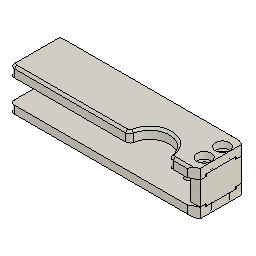
Summit (Autodesk Fusion 360 design; units mm, degrees)
Autodesk Fusion 360 part; units mm, degrees
sketch "Faceplate_Profile" plane through (0, 0, 0) normal (0, 0, 1) x (1, 0, 0)
  line L0 (0, 0) -> (85, 0)
  line L1 (85, 0) -> (85, 23)
  line L2 (85, 23) -> (0, 23)
  line L3 (0, 23) -> (0, 0)
  arc A0 (72.75, 0) -> (54.75, 0) centre (63.75, 0.1978) ccw
  line L4 (63.75, 0.1978) -> (63.75, 9.2) construction
  circle A1 centre (88, 11.5) radius 12 construction
  line L5 (85, 11.5) -> (88, 11.5) construction
  line L6 (80.7138, 21.0347) -> (80.7138, 1.9653)
  line L7 (80.7138, 1.9653) -> (89.4835, -4.7363) construction
  line L8 (80.7138, 21.0347) -> (88.5708, 27.0388) construction
  arc A2 (80.7138, 21.0347) -> (80.7138, 1.9653) centre (88, 11.5) ccw
  line L9 (84.2138, 26.5305) -> (84.2138, -3.5305) construction
  arc A3 (84.2138, 26.5305) -> (84.2138, -3.5305) centre (88, 11.5) ccw construction
  line L10 (72.5, 23) -> (72.5, 0) construction
  line L11 (80.7138, 1.9653) -> (72.5, 1.9653)
  line L12 (72.5, 1.9653) -> (72.5, 21.0347)
  line L13 (72.5, 21.0347) -> (80.7138, 21.0347)
  line L14 (80.7138, 21.0347) -> (80.7138, 1.9653)
  circle A4 centre (70.5, 11.5) radius 2
  line L15 (80.7138, 21.0347) -> (85, 21.0347)
  line L16 (80.7138, 1.9653) -> (85, 1.9653)
  dimension "d12" = 85
  dimension "d13" = 23
  dimension "d14" = 9.2
  dimension "d16" = 63.75
  dimension "d17" = 18
  dimension "d42" = 24
  dimension "d43" = 3
  dimension "d44" = 3.5
  dimension "d45" = 4
  constraint horizontal L0
  constraint vertical L1
  constraint horizontal L2
  constraint vertical L3
  constraint coincident L0.start L3.end
  constraint coincident L0 A0.end
  constraint coincident L0 A0.start
  constraint coincident A0.centre L4.start
  constraint midpoint A0 L4.end
  constraint midpoint L1 L5.start
  constraint coincident A1.centre L5.end
  constraint horizontal L5
  constraint coincident A1 L6.start
  constraint coincident A1 L6.end
  constraint vertical L6
  constraint tangent A1 L8
  constraint tangent A1 L7
  constraint tangent L7 A2
  constraint coincident L2 L10.start
  constraint coincident L0 L10.end
  constraint perpendicular L0 L10
  constraint horizontal L11
  constraint vertical L12
  constraint horizontal L13
  constraint vertical L14
  constraint tangent L12 A4
  constraint coincident L1 L15.end
  constraint perpendicular L1 L15
  constraint perpendicular L6 L16
  measures "d12" distance of L0.start L0.end
  measures "d13" distance of L0.start L2.end
  measures "d14" distance of L0 L4.end
  measures "d16" horizontal distance of L0.start A0.centre
  measures "d17" distance of A0.end A0.start
  measures "d42" diameter of A1
  measures "d43" distance of L1 A1.centre
  measures "d45" diameter of A4
extrude "Extrude1" add sketch "Faceplate_Profile" along normal blind 4.6 contours A4 | L0 L1 L2 L3 A0 L12 L13 L15 | L0 L1 A0 L11 L16 | A0 A2 L11 L12 L13 | L1 L6 L14 L15 L16 | L6 A2 L14 makes body 1 in component "Plate_Top"
extrude "Extrude1'" add sketch "Faceplate_Profile" against normal blind 4.6 from surface at -10.8 separate body contours A4 | L0 L1 L2 L3 A0 L12 L13 L15 | L0 A0 L11 L12 | L0 L1 A0 L11 L16 | A0 A2 L11 L12 L13 | A0 L11 L12 | L1 L6 L14 L15 L16 | L6 A2 L14 makes body 2 in component "Plate_Bottom"
extrude "Extrude1''" add sketch "Faceplate_Profile" against normal up to surface (10.8 mm away) separate body contours A4 | L1 L6 L14 L15 L16 | L6 A2 L14 makes body 3 at (76.9486, 16.1761, -7.2) makes body 4 at (69.1766, 12.9996, -7.2) in component "Ring_Holder"
sketch "Holder things" plane through (0, 0, -10.8) normal (0, 0, 1) x (-1, 0, 0) in component "Ring_Holder"
  line L0 (-85, 0) -> (-85, -23)
  line L1 (-85, -23) -> (0, -23)
  line L2 (0, -23) -> (0, 0)
  line L3 (0, 0) -> (-85, 0)
  arc A0 (-80.7138, -21.0347) -> (-80.7138, -1.9653) centre (-88, -11.5) ccw
  line L4 (-80.7138, -1.9653) -> (-85, -1.9653)
  line L5 (-85, -1.9653) -> (-85, -21.0347)
  line L6 (-85, -21.0347) -> (-80.7138, -21.0347)
  circle A1 centre (-70.5, -11.5) radius 2
  line L7 (0, 0) -> (-85, 0)
  line L8 (-85, 0) -> (-85, -23)
  line L9 (0, -23) -> (0, 0)
  line L10 (-85, -23) -> (0, -23)
  line L11 (-78.0788, -18.2506) -> (-78.0788, -4.7494)
  line L12 (-78.0788, -4.7494) -> (-85, -4.7494)
  line L13 (-85, -4.7494) -> (-85, -18.2506)
  line L14 (-85, -18.2506) -> (-78.0788, -18.2506)
  circle A2 centre (-81.5394, -7.2929) radius 1.5
  circle A3 centre (-81.5394, -15.7071) radius 1.5
  line L15 (-81.5394, -7.2929) -> (-81.5394, -15.7071) construction
  line L16 (-78.0788, -11.5) -> (-85, -11.5) construction
  circle A4 centre (-70.5, -11.5) radius 1.5
  point P0 (-70.5, -11.5)
  dimension "d48" = 3
  dimension "d49" = 3
  dimension "d50" = 3
  constraint perpendicular L11 L12
  constraint parallel L11 L13
  constraint parallel L12 L14
  constraint coincident A0 L11.end
  constraint vertical L11
  constraint coincident A0 L11.start
  constraint coincident A2.centre L15.start
  constraint coincident A3.centre L15.end
  constraint vertical L15
  constraint midpoint L11 L16.start
  constraint midpoint L5 L16.end
  constraint midpoint L15 L16
  constraint coincident P0 A1.centre
  measures "d48" diameter of A2
  measures "d49" diameter of A3
  measures "d50" diameter of A4
extrude "Extrude2" cut sketch "Holder things" along normal blind -1 and the other way blind 0 contours L0 L5 L8 L11 L12 L13 L14 | A2 | A3 bodies 2 in component "Plate_Bottom"
extrude "Extrude2'" cut sketch "Holder things" along normal blind 1 from surface at 10.8 contours L0 L5 L8 L11 L12 L13 L14 | A2 | A3 bodies 1 in component "Plate_Top"
extrude "Extrude2''" add sketch "Holder things" against normal blind 1 contours L0 L5 L8 L11 L12 L13 L14 bodies 3 in component "Ring_Holder"
extrude "Extrude3" add sketch "Holder things" along normal blind 1 from surface at 10.8 contours L0 L5 L8 L11 L12 L13 L14 bodies 3 in component "Ring_Holder"
move_face "OffsetFaces1" offset -0.2 3 faces at (82.6929, 18.2506, -11.1333) (80.3859, 4.7494, -11.1333) (78.0788, 13.7502, -11.1333) on bodies 2 in component "Plate_Bottom"
move_face "OffsetFaces1'" offset -0.2 3 faces at (78.0788, 13.7502, 0.3333) (82.6929, 18.2506, 0.3333) (80.3859, 4.7494, 0.3333) on bodies 1 in component "Plate_Top"
sketch "D_plate_bores" plane through (0, 0, 4.6) normal (0, 0, 1) x (-1, 0, 0) in component "Ring_Holder"
  line L0 (-85, 0) -> (-85, -23)
  line L1 (-85, -23) -> (0, -23)
  line L2 (0, -23) -> (0, 0)
  line L3 (0, 0) -> (-54.75, 0)
  arc A0 (-72.75, 0) -> (-54.75, 0) centre (-63.75, -0.1978) ccw
  line L4 (-72.75, 0) -> (-85, 0)
  circle A1 centre (-70.5, -11.5) radius 2
  circle A2 centre (-70.5, -11.5) radius 2
  line L5 (-85, -4.7494) -> (-85, -18.2506)
  line L6 (-85, -18.2506) -> (-78.0788, -18.2506)
  line L7 (-78.0788, -18.2506) -> (-78.0788, -4.7494)
  line L8 (-78.0788, -4.7494) -> (-85, -4.7494)
  circle A3 centre (-81.5394, -15.7071) radius 1.5
  circle A4 centre (-81.5394, -7.2929) radius 1.5
hole "Hole1" at (81.5394, 7.2929, 4.6) at (81.5394, 15.7071, 4.6) direction (0, 0, -1) diameter 3.4 depth 19 tip angle 180 counterbore diameter 6.5 counterbore depth 3 bodies 1 in component "Plate_Top"
hole "Hole1'" at (81.5394, 7.2929, 4.6) at (81.5394, 15.7071, 4.6) direction (0, 0, -1) diameter 3.4 depth 19 tip angle 180 counterbore diameter 6.5 counterbore depth 3 bodies 2 in component "Plate_Bottom"
hole "Hole1''" at (81.5394, 7.2929, 4.6) at (81.5394, 15.7071, 4.6) direction (0, 0, -1) diameter 3.4 depth 19 tip angle 180 counterbore diameter 6.5 counterbore depth 3 bodies 3 in component "Ring_Holder"
sketch "D_plate_nuts" plane through (0, 0, -15.4) normal (0, 0, 1) x (-1, 0, 0) in component "Plate_Bottom"
  circle A0 centre (-70.5, -11.5) radius 2
  circle A1 centre (-81.5394, -15.7071) radius 1.5
  circle A2 centre (-81.5394, -7.2929) radius 1.5
  circle A3 centre (-70.5, -11.5) radius 2
  line L0 (0, 0) -> (0, -23)
  line L1 (0, -23) -> (-85, -23)
  line L2 (-85, -23) -> (-85, 0)
  line L3 (-85, 0) -> (0, 0)
  line L4 (-83.2137, -4.3929) -> (-84.888, -7.2929)
  line L5 (-84.888, -7.2929) -> (-83.2137, -10.1929)
  line L6 (-83.2137, -10.1929) -> (-79.8651, -10.1929)
  line L7 (-79.8651, -10.1929) -> (-78.1908, -7.2929)
  line L8 (-78.1908, -7.2929) -> (-79.8651, -4.3929)
  line L9 (-79.8651, -4.3929) -> (-83.2137, -4.3929)
  line L10 (-84.888, -15.7071) -> (-83.2137, -18.6071)
  line L11 (-83.2137, -18.6071) -> (-79.8651, -18.6071)
  line L12 (-79.8651, -18.6071) -> (-78.1908, -15.7071)
  line L13 (-78.1908, -15.7071) -> (-79.8651, -12.8071)
  line L14 (-79.8651, -12.8071) -> (-83.2137, -12.8071)
  line L15 (-83.2137, -12.8071) -> (-84.888, -15.7071)
  point P0 (-81.5394, -7.2929)
  point P1 (-81.5394, -15.7071)
  dimension "d81" = 2.9
  dimension "d82" = 2.9
  constraint coincident P0 A2.centre
  constraint horizontal L9
  constraint coincident P1 A1.centre
  constraint horizontal L14
  measures "d81" distance of P0 L9
  measures "d82" distance of P1 L15
extrude "Extrude3'" cut sketch "D_plate_nuts" along normal blind 2.8 from surface at 0.8 contours A1 | A2 | L4 L5 L6 L7 L8 L9 | L10 L11 L12 L13 L14 L15 bodies 2 in component "Plate_Bottom"
hole "Hole2" at (70.5, 11.5, -15.4) direction (0, 0, 1) diameter 3.2 depth 19.2 tip angle 180 counterbore diameter 6.5 counterbore depth 1.8 bodies 1 in component "Plate_Top"
hole "Hole2'" at (70.5, 11.5, -15.4) direction (0, 0, 1) diameter 3.2 depth 19.2 tip angle 180 counterbore diameter 6.5 counterbore depth 1.8 bodies 2 in component "Plate_Bottom"
hole "Hole2''" at (70.5, 11.5, -15.4) direction (0, 0, 1) diameter 3.2 depth 19.2 tip angle 180 counterbore diameter 6.5 counterbore depth 1.8 bodies 4 in component "Ring_Holder"
fillet "Fillet1" radius 2 2 edges at (0, 23, -13.1) (0, 0, -13.1) on bodies 2 in component "Plate_Bottom"
fillet "Fillet1'" radius 2 4 edges at (54.75, 0, 2.3) (72.75, 0, 2.3) (0, 0, 2.3) (0, 23, 2.3) on bodies 1 in component "Plate_Top"
chamfer "Chamfer1" distance 4 distance2 2 1 edges at (85, 23, -13.1) measured on face at (29.6667, 23, -13.8667) on bodies 2 in component "Plate_Bottom"
chamfer "Chamfer1" distance 2 distance2 4 1 edges at (85, 0, -13.1) measured on face at (85, 13.8169, -14.2) on bodies 2 in component "Plate_Bottom"
chamfer "Chamfer1" distance 1 distance2 1 5 edges at (43.5, 0, -15.4) (0.5858, 0.5858, -15.4) (0, 11.5, -15.4) (0.5858, 22.4142, -15.4) (43.5, 23, -15.4) measured on face at (23.753, 11.581, -15.4) measured on face at (1.9048, 0.0023, -13.8667) measured on face at (23.753, 11.581, -15.4) measured on face at (0.0023, 21.0952, -13.8667) measured on face at (23.753, 11.581, -15.4) on bodies 2 in component "Plate_Bottom"
chamfer "Chamfer1'" distance 4 distance2 2 1 edges at (85, 0, 2.3) measured on face at (78.069, 0, 1.5333) on bodies 1 in component "Plate_Top"
chamfer "Chamfer1'" distance 2 distance2 4 1 edges at (85, 23, 2.3) measured on face at (85, 13.7502, 3.4) on bodies 1 in component "Plate_Top"
chamfer "Chamfer1'" distance 1 distance2 1 9 edges at (27.4482, 0, 4.6) (54.1896, 0.4744, 4.6) (63.75, 9.2, 4.6) (73.3104, 0.4744, 4.6) (79.8018, 0, 4.6) (43.5, 23, 4.6) (0.5858, 22.4142, 4.6) (0, 11.5, 4.6) (0.5858, 0.5858, 4.6) measured on face at (18.9655, 7.6667, 4.6) measured on face at (53.8826, 0.26, 1.5333) measured on face at (18.9655, 7.6667, 4.6) measured on face at (73.7, 0.2157, 1.5333) measured on face at (18.9655, 7.6667, 4.6) measured on face at (18.9655, 7.6667, 4.6) measured on face at (0.0023, 21.0952, 1.5333) measured on face at (18.9655, 7.6667, 4.6) measured on face at (1.9048, 0.0023, 1.5333) on bodies 1 in component "Plate_Top"
component "Plate_Top" placed x (1, 0, 0) y (0, 1, 0) z (0, 0, 1) at (0, 0, 0)
component "Plate_Bottom" placed x (1, 0, 0) y (0, 1, 0) z (0, 0, 1) at (0, 0, 0)
component "Ring_Holder" placed x (1, 0, 0) y (0, 1, 0) z (0, 0, 1) at (0, 0, 0)
equation "Key_Length = 70 mm" comment "Max length of key"
equation "Key_Width = 28 mm" comment "Max width of key"
equation "Key_Thicc = 2,8 mm" comment "Max thickness of key"
equation "Case_Width = Key_Width - 5 mm" comment "Full width of case"
equation "Case_Length = Key_Length + 15 mm" comment "Full length of case"
equation "Plate_Thicc = 4,6 mm" comment "Thickness of each case plate"
equation "Plate_Spacing = ( ( Key_Thicc + 0,6 mm ) * Key_Count ) + 0,6 mm" comment "Full extent of space that will accomodate the keys"
equation "Key_Count = 3" comment "Number of keys to fit inside keyring"
equation "Finger_indent = Case_Width * 2 / 5"
equation "Ring_ID = 24 mm" comment "Inner Diameter of keychain ring"
equation "Ring_Thickness = 3 mm"
equation "d12 = Case_Length"
equation "d13 = Case_Width"
equation "d14 = Finger_indent"
equation "d16 = ( Case_Length * 3 / 4 mm ) * 1 mm"
equation "d18 = Plate_Thicc"
equation "d23 = -Plate_Spacing"
equation "d24 = -Plate_Thicc"
equation "d42 = Ring_ID"
equation "d43 = Ring_ID / 8"
equation "d44 = Ring_Thickness + 0,5 mm"
equation "d51 = -Plate_Thicc + 3,6 mm"
equation "d56 = -d51"
equation "d58 = d51"
equation "d61 = -d51"
equation "d77 = 2 * Plate_Thicc + Plate_Spacing - 1 mm"
equation "d78 = 2 * Plate_Thicc + Plate_Spacing - 1 mm"
equation "d79 = 2 * Plate_Thicc + Plate_Spacing - 1 mm"
equation "d81 = ( 5,8 / 2 ) * 1 mm"
equation "d82 = ( 5,8 / 2 ) * 1 mm"
equation "d86 = 2 * Plate_Thicc + Plate_Spacing - 0,8 mm"
equation "d91 = 2 * Plate_Thicc + Plate_Spacing - 0,8 mm"
equation "d96 = 2 * Plate_Thicc + Plate_Spacing - 0,8 mm"
named bodies: "D_Plate", "Standoff"
